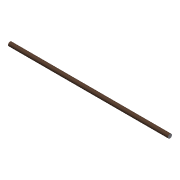
# Autodesk Inventor part: 2p3reb
Saved by Autodesk Inventor 2016 (Build 200138000, 138)
## iProperties
Company: HERA Project
Created: 2013-05-20
Part Number: 2p3reb
Material: Steel, Mild
Document SubType Name: Modeling
Designer: David DeBoer
Density: 7.86 g/cm^3
Description: Support stand rebar
Mass: 127.463 g
Surface Area: 86.0389 cm^2
Volume: 16.2167 cm^3
Appearance: Steel
Author: David DeBoer
Title: Support stand rebar
Autodesk Inventor part; units mm, degrees
ref_plane "YZ Plane" through (0, 0, 0) normal (1, 0, 0) x (0, 1, 0)
ref_plane "XZ Plane" through (0, 0, 0) normal (0, 1, 0) x (-1, 0, 0)
ref_plane "XY Plane" through (0, 0, 0) normal (0, 0, 1) x (1, 0, 0)
sketch "Sketch2" plane through (0, 0, 0) normal (1, 0, 0) x (0, 1, 0)
  circle A0 centre (0, 0) radius 3.81
  dimension "d3" = 7.62
  constraints: 1 centre point, 1 coincident
  measures "d3" diameter of A0
extrude "Extrusion2" add sketch "Sketch2" along normal blind 300
body "Solid2"
